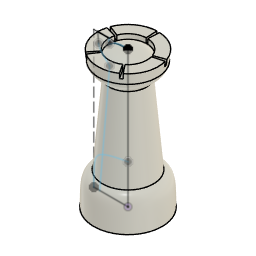
Rook v2 (Autodesk Fusion 360 design; units mm, degrees)
Autodesk Fusion 360 part; units mm, degrees
sketch "Sketch1" plane through (0, 0, 0) normal (0, 1, 0) x (1, 0, 0)
  line L0 (0, 0) -> (0, -70)
  line L1 (0, 0) -> (-17.5, 0)
  spline S0 degree 5 poles (-17.5, 0) (-17.5, -1.949) (-17.4812, -5.4749) (-17.3967, -9.6483) (-17.034, -13.32) (-15.2217, -16.0242) (-11.5143, -17.5778) (-6.6893, -18.7492) (-2.4074, -19.5755) (0, -20) knots 0 0 0 0 0 0 0.2 0.4 0.6 0.8 1 1 1 1 1 1
  line L2 (-5, -19.1184) -> (5, -20.8816)
  line L3 (-17.5, 4) -> (-17.5, -4)
  line L4 (-14.4973, 0) -> (-9.4367, -57.843)
  spline S1 degree 5 poles (-9.4367, -57.843) (-9.7977, -58.204) (-10.4974, -58.8976) (-11.4805, -59.8532) (-12.6619, -60.9863) (-13.8936, -62.2839) (-14.6089, -63.319) (-14.9312, -64.1356) (-15.0367, -64.7042) (-15.0621, -64.9946) knots 0 0 0 0 0 0 0.2 0.4 0.6 0.8 1 1 1 1 1 1
  line L5 (-15.0621, -64.9946) -> (-15.5, -70)
  line L6 (-14.9783, -64.0369) -> (-15.1459, -65.9522)
  line L7 (-17.5, -70) -> (0, -70) construction
  line L8 (-15.5, -70) -> (-9.7348, -70)
  line L9 (-9.7348, -70) -> (-9.7348, -67.5)
  line L10 (-8.1537, -56.5599) -> (-10.7198, -59.1261)
  line L11 (-17.5, 0) -> (-17.5, -70) construction
  spline S2 degree 5 poles (-9.7348, -67.5) (-9.5938, -67.5) (-9.3202, -67.5511) (-8.9352, -67.7806) (-8.3991, -68.3325) (-7.2315, -69.1675) (-5.359, -69.7194) (-3.0799, -69.9489) (-1.103, -70) (0, -70) knots 0 0 0 0 0 0 0.2 0.4 0.6 0.8 1 1 1 1 1 1
  line L12 (-10.1589, -67.5) -> (-9.3107, -67.5)
  line L13 (-3.3162, -70) -> (3.3162, -70)
  dimension "d1" = 70
  dimension "d2" = 17.5
  dimension "d3" = 5
  dimension "d4" = 45
  dimension "d5" = 5
  dimension "d6" = 10
  dimension "d14" = 2.5
  dimension "d15" = 2
  constraint coincident L0.start L1.start
  constraint vertical L0
  constraint perpendicular L0 L1
  constraint midpoint L2 S0.end
  constraint midpoint L1.end L3
  constraint vertical L3
  constraint midpoint S1.end L6
  constraint parallel L5 L6
  constraint coincident L7 L8.end
  constraint perpendicular L8 L9
  constraint midpoint L4.end L10
  constraint vertical L11
  constraint horizontal L7
  constraint coincident L0 S0.end
  constraint coincident L1 L4.start
  constraint midpoint L9.end L12
  constraint perpendicular L9 L12
  constraint midpoint L0.end L13
  constraint perpendicular L0 L13
  constraint perpendicular L7 L9
  measures "d1" distance of L0.start L0.end
  measures "d2" distance of L0.start L1.end
  measures "d3" angle of L0 L5
  measures "d4" angle of L0 L10
  measures "d5" angle of L0 L4
  measures "d6" angle of L1 L2
  measures "d14" distance of L8.end L9.end
  measures "d15" distance of L5.end L7.start
revolve "Revolve1" add sketch "Sketch1" angle 360 about axis through (0, 0, 0) along (0, 0, 1)
sketch "Sketch3" plane through (0, 0, 70) normal (0, 0, 1) x (-1, 0, 0)
  circle A0 centre (0, 0) radius 9.7348
  circle A1 centre (0, 0) radius 15.5
  line L0 (0, 0) -> (0.6761, -15.4852)
  line L1 (0, 0) -> (-0.6761, -15.4852)
  line L2 (0, 0) -> (0, -15.5) construction
  dimension "d8" = 5
  dimension "d9" = 2.5
  constraint coincident A0.centre A1.centre
  constraint coincident A1 L0.end
  constraint coincident A1 L1.end
  constraint coincident A1 L2.end
  measures "d8" angle of L0 L1
  measures "d9" angle of L1 L2
extrude "Extrude1" cut sketch "Sketch3" against normal up to surface (2.5 mm away) contours A0 A1 L0 L1 picked at (0.4421, -13.5697)
pattern_circular "C-Pattern1" count 5 over 360 about axis through (0, 0, 1.75) along (0, 0, 1) of "Extrude1"
equation "d2 = 3.5 cm / 2"
